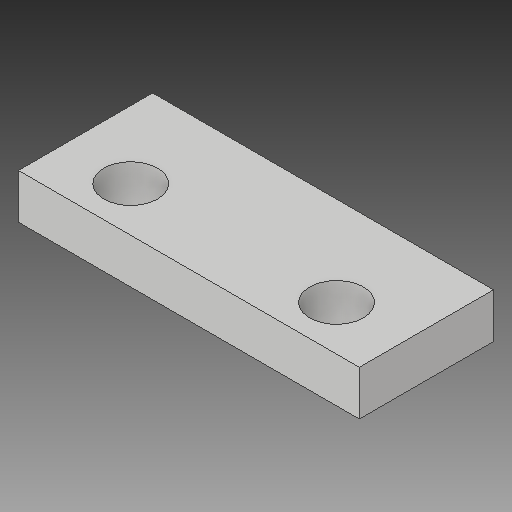
# Autodesk Inventor part: SuporteGuiasCabeçasAquecimento
Saved by Autodesk Inventor 2018 (Build 220112000, 112)
## iProperties
Created: 2018-07-23
Part Number: SuporteGuiasCabeçasAquecimento
Material: Genérico
Document SubType Name: Modeling
Designer: Usuario
Density: 1 g/cm^3
Appearance: Padrão
Mass: 20.6392 g
Surface Area: 70.0335 cm^2
Volume: 20.6392 cm^3
Author: Usuario
Autodesk Inventor part; units mm, degrees
ref_plane "YZ Plane" through (0, 0, 0) normal (1, 0, 0) x (0, 1, 0)
ref_plane "XZ Plane" through (0, 0, 0) normal (0, 1, 0) x (-1, 0, 0)
ref_plane "XY Plane" through (0, 0, 0) normal (0, 0, 1) x (1, 0, 0)
sketch "Esboço1" plane through (0, 0, 0) normal (0, 0, 1) x (1, 0, 0)
  line L0 (-34.4331, 101.047) -> (41.7669, 101.047)
  line L1 (41.7669, 101.047) -> (41.7669, 91.027)
  line L2 (41.7669, 91.027) -> (-34.4331, 91.027)
  line L3 (-34.4331, 91.027) -> (-34.4331, 101.047)
  point P0 (0, 0)
  dimension "d0" = 76.2
  dimension "d1" = 10.02
  constraints: 8 end point, 2 parallel, 1 horizontal, 1 perpendicular
  measures "d0" distance of L1.end L2.end
  measures "d1" distance of L0.end L1.end
extrude "Extrusão1" add sketch "Esboço1" along normal blind 30
sketch "Esboço2" plane through (-34.4331, 101.047, 0) normal (0, 1, 0) x (1, 0, 0)
  line L0 (76.2, 0) -> (76.2, -30) projected
  line L1 (76.2, -20) -> (0, -20)
  line L2 (0, 0) -> (0, -30) projected
  line L3 (0, 0) -> (76.2, 0) projected
  line L4 (38.1, -40) -> (38.1, 0)
  circle A0 centre (61.1, -20) radius 6.7139
  circle A1 centre (15.1, -20) radius 6.7459
  point P0 (34.4331, 0)
  dimension "d4" = 20
  dimension "d5" = 23
  dimension "d6" = 23
  constraints: 4 end point, 4 point on line, 2 centre point, 1 horizontal, 1 midpoint
  measures "d4" distance between parallel lines of L3 L1
  measures "d5" distance from line of A0.centre L4
  measures "d6" distance from line of L4 A1.centre
hole "Furo1" at (26.6669, 101.047, 20) at (-19.3331, 101.047, 20) direction (0, -1, 0) diameter 12 end through all
equation "\"d6\" = d5"
equation "\"d12\" = 0.5 * d1"
